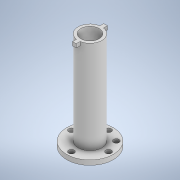
# Autodesk Inventor part: Base
Saved by Autodesk Inventor 2022 (Build 260153000, 153)
## iProperties
Created: 2022-08-24
Part Number: Base
Material: Generic
Document SubType Name: Modeling
Designer: Usuario
Density: 1 g/cm^3
Appearance: Default
Author: Usuario
Autodesk Inventor part; units mm, degrees
ref_plane "YZ Plane" through (0, 0, 0) normal (1, 0, 0) x (0, 1, 0)
ref_plane "XZ Plane" through (0, 0, 0) normal (0, 1, 0) x (-1, 0, 0)
ref_plane "XY Plane" through (0, 0, 0) normal (0, 0, 1) x (1, 0, 0)
sketch "Sketch1" plane through (0, 0, 0) normal (0, 1, 0) x (-1, 0, 0)
  circle A0 centre (0, 0) radius 9.75
  circle A1 centre (0, 0) radius 12.75
  dimension "d0" = 19.5
  dimension "d1" = 3
  constraints: 2 centre point, 2 coincident
  measures "d0" diameter of A0
  measures "d1" radial gap between concentric circles of A0 A1
extrude "Extrusion1" add sketch "Sketch1" along normal blind 100
sketch "Sketch2" plane through (0, 0, 0) normal (0, -1, 0) x (1, 0, 0)
  circle A0 centre (0, 0) radius 5
  circle A1 centre (0, 0) radius 7
  dimension "d4" = 10
  dimension "d5" = 14
  constraints: 2 centre point, 2 coincident
  measures "d4" diameter of A0
  measures "d5" diameter of A1
extrude "Extrusion2" add sketch "Sketch2" against normal blind 2
sketch "Sketch3" plane through (0, 0, 0) normal (0, -1, 0) x (1, 0, 0)
  circle A0 centre (0, 0) radius 12.75
  constraints: 1 centre point, 1 coincident
extrude "Extrusion3" add sketch "Sketch3" along normal blind 5
sketch "Sketch4" plane through (0, -5, 0) normal (0, -1, 0) x (1, 0, 0)
  circle A0 centre (0, 0) radius 25
  circle A1 centre (0, 0) radius 7 projected
  circle A2 centre (0, 0) radius 20
  circle A3 centre (-20, 0) radius 3
  circle A4 centre (0, 20) radius 3
  circle A5 centre (20, 0) radius 3
  circle A6 centre (0, -20) radius 3
  circle A7 centre (0, 0) radius 12.75 projected
  line L0 (-20, 0) -> (0, 0)
  circle A8 centre (0, 0) radius 9.75 projected
  line L1 (0, 20) -> (0, 0)
  circle A9 centre (0, 0) radius 5 projected
  line L2 (20, 0) -> (0, 0)
  line L3 (0, -20) -> (0, 0)
  circle A10 centre (14.1421, -14.1421) radius 3
  line L4 (14.1421, -14.1421) -> (0, 0)
  line L5 (-35, 0) -> (35, 0) projected
  dimension "d10" = 50
  dimension "d11" = 40
  dimension "d12" = 90
  dimension "d13" = 90
  dimension "d14" = 90
  dimension "d15" = 45
  dimension "d16" = 6
  constraints: 10 end point, 7 centre point, 5 point on circle, 4 equal radius, 2 coincident, 1 point on line
  measures "d10" diameter of A0
  measures "d11" diameter of A2
  measures "d12" angle of L2 L1
  measures "d13" angle of L0 L1
  measures "d14" angle of L3 L0
  measures "d15" angle of L3 L4
  measures "d16" diameter of A4
extrude "Extrusion4" add sketch "Sketch4" against normal blind 5 contours L5 A5 A2 A4 A3 A0 | A0 L5 A3 A2 A6 A10 A5 | A5 L2 A7 L1 A4 A2 | A2 A10 L4 A7 L2 A5 | A2 A4 L1 A7 L0 A3 | A3 L0 A7 L3 A6 A2 | L2 A8 L1 A7 | A7 L4 A8 L2 | A10 A2 A6 L3 A7 L4 | L0 A8 L3 A7 | A7 L1 A8 L0 | A7 L3 A8 L4 | L2 A1 L1 A8 | A8 L4 A1 L2 | A8 L1 A1 L0 | L0 A1 L3 A8 | A8 L3 A1 L4 | L2 A9 L1 A1 | A1 L4 A9 L2 | L0 A9 L3 A1 | A1 L1 A9 L0 | A1 L3 A9 L4 | L2 L1 A9 | A9 L4 L2 | A9 L1 L0 | L0 L3 A9 | A9 L3 L4
sketch "Sketch5" plane through (0, 100, 0) normal (0, 1, 0) x (1, 0, 0)
  circle A0 centre (0, 0) radius 12.75 projected
  circle A1 centre (0, 0) radius 9.75 projected
  line L0 (1.9927, -8.75) -> (-2.0073, -8.75)
  line L1 (-2.0073, -8.75) -> (-2.0073, -16.75)
  line L2 (-2.0073, -16.75) -> (1.9927, -16.75)
  line L3 (1.9927, -16.75) -> (1.9927, -8.75)
  circle A2 centre (0, 0) radius 12.75 projected
  line L4 (1.9927, -8.75) -> (-2.0073, -16.75) construction
  line L5 (-2.0073, -8.75) -> (1.9927, -16.75) construction
  line L6 (1.9927, 8.75) -> (-2.0073, 8.75)
  line L7 (-2.0073, 8.75) -> (-2.0073, 16.75)
  line L8 (-2.0073, 16.75) -> (1.9927, 16.75)
  line L9 (1.9927, 16.75) -> (1.9927, 8.75)
  line L10 (1.9927, 8.75) -> (-2.0073, 16.75) construction
  line L11 (-2.0073, 8.75) -> (1.9927, 16.75) construction
  point P0 (-0.0073, -12.75)
  point P1 (-0.0073, 12.75)
  point P2 (1.9927, -12.5933)
  point P3 (-2.0073, -12.591)
  point P4 (-2.0073, 12.591)
  point P5 (1.9927, 12.5933)
  dimension "d19" = 4
  dimension "d20" = 8
  constraints: 24 end point, 4 midpoint, 4 parallel, 2 equal length, 2 horizontal, 2 perpendicular, 1 point on line, 4 other
  measures "d19" distance of L7.end L8.end
  measures "d20" distance of L6.end L7.end
extrude "Extrusion5" add sketch "Sketch5" against normal blind 4 contours A0 L7 L8 L9 | L3 L2 L1 A0
body "Solid1"
